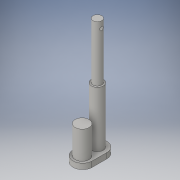
# Autodesk Inventor part: Linear Actuator
Saved by Autodesk Inventor 2016 (Build 200138000, 138)
## iProperties
Created: 2015-12-05
Part Number: Linear Actuator
Material: Generic
Document SubType Name: Modeling
Designer: Javier
Density: 1 g/cm^3
Appearance: Default
Author: Javier
Autodesk Inventor part; units mm, degrees
ref_plane "YZ Plane" through (0, 0, 0) normal (1, 0, 0) x (0, 1, 0)
ref_plane "XY Plane" through (0, 0, 0) normal (0, 0, 1) x (1, 0, 0)
sketch "Sketch1" plane through (0, 0, 0) normal (0, 1, 0) x (-1, 0, 0)
  circle A0 centre (0, 0) radius 10.795
  circle A1 centre (0, 37.7825) radius 10.795
  dimension "d11" = 21.59
  constraints: 2 centre point, 1 coincident
  measures "d11" diameter of A0
extrude "Extrusion1" add sketch "Sketch1" along normal blind 101.6 contours A0
sketch "Sketch2" plane through (0, 0, 0) normal (0, 1, 0) x (-1, 0, 0)
  circle A0 centre (0, 27.7858) radius 12.7
  point P0 (0, 0)
  dimension "d2" = 25.4
  constraints: 1 centre point
  measures "d2" diameter of A0
extrude "Extrusion2" add sketch "Sketch2" along normal blind 50.8
sketch "Sketch3" plane through (0, 0, 0) normal (0, 1, 0) x (-1, 0, 0)
  arc A0 (17.4625, 26.9867) -> (-17.4625, 28.5282) centre (-0.0401, 26.849) ccw
  arc A1 (-17.4625, 0) -> (17.4625, 0) centre (0, 0) ccw
  line L0 (17.4625, 0) -> (17.4625, 26.9867)
  line L1 (-17.4625, 0) -> (-17.4625, 28.5282)
  constraints: 4 end point, 4 point on circle, 2 centre point, 2 vertical, 1 coincident
extrude "Extrusion3" add sketch "Sketch3" against normal blind 10.16
sketch "Sketch4" plane through (0, 0, 0) normal (0, 1, 0) x (-1, 0, 0)
  point P0 (0, 0)
ref_plane "Work Plane1" through (0, 101.6, 0) normal (0, 1, 0) x (-1, 0, 0)
sketch "Sketch5" plane through (0, 101.6, 0) normal (0, 1, 0) x (-1, 0, 0)
  circle A0 centre (0, 0) radius 7.9375
  dimension "d8" = 15.875
  constraints: 1 centre point, 1 coincident
  measures "d8" diameter of A0
extrude "Extrusion4" add sketch "Sketch5" along normal blind 101.6
sketch "Sketch6" plane through (0, 0, 0) normal (1, 0, 0) x (0, 1, 0)
  circle A0 centre (190.95, 0) radius 3.25
  line L0 (203.2, -7.9375) -> (203.2, 7.9375) projected
  line L1 (203.2, -7.9375) -> (203.2, 7.9375)
  point P0 (0, 0)
  dimension "d14" = 6.5
  dimension "d15" = 12.25
  constraints: 2 end point, 1 centre point, 1 vertical
  measures "d14" diameter of A0
  measures "d15" distance from line of A0.centre L0
extrude "Extrusion5" cut sketch "Sketch6" along normal mid plane 101.6
body "Solid1"
